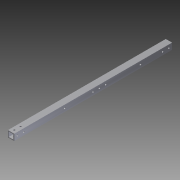
# Autodesk Inventor part: towermediumfrontthing
Saved by Autodesk Inventor 2011 SP1 (Build 150282100, 282)
## iProperties
Created: 2012-01-18
Part Number: towermediumfrontthing
Document SubType Name: Modeling
Designer: Christopher
Density: 1 g/cm^3
Author: Christopher
Autodesk Inventor part; units mm, degrees
ref_plane "YZ Plane" through (0, 0, 0) normal (1, 0, 0) x (0, 1, 0)
ref_plane "XZ Plane" through (0, 0, 0) normal (0, 1, 0) x (-1, 0, 0)
ref_plane "XY Plane" through (0, 0, 0) normal (0, 0, 1) x (1, 0, 0)
sketch "Sketch1" plane through (0, 0, 0) normal (0, 0, 1) x (1, 0, 0)
  line L0 (0, 0) -> (25.4, 0)
  line L1 (25.4, 0) -> (25.4, 25.4)
  line L2 (25.4, 25.4) -> (0, 25.4)
  line L3 (0, 25.4) -> (0, 0)
  line L4 (3.175, 3.175) -> (22.225, 3.175)
  line L5 (22.225, 3.175) -> (22.225, 22.225)
  line L6 (22.225, 22.225) -> (3.175, 22.225)
  line L7 (3.175, 22.225) -> (3.175, 3.175)
  dimension "d0" = 25.4
  dimension "d1" = 25.4
  dimension "d2" = 3.175
  constraints: 16 end point, 4 parallel, 2 perpendicular, 1 horizontal, 3 other
  measures "d0" distance of L1.end L2.end
  measures "d1" distance of L0.end L1.end
  measures "d2" distance between parallel lines of L3 L7
extrude "Extrusion1" add sketch "Sketch1" against normal blind 635
sketch "Sketch3" plane through (0, 25.4, 0) normal (0, 1, 0) x (1, 0, 0)
  line L0 (25.4, 0) -> (0, 0) projected
  point P0 (12.7, 12.7)
  point P1 (12.7, 38.1)
  dimension "d24" = 12.7
  dimension "d25" = 25.4
  measures "d24" distance from line of L0 point (12.7, 12.7)
  measures "d25" distance of point (12.7, 38.1) point (12.7, 12.7)
hole "Hole3" at (12.7, 25.4, -12.7) at (12.7, 25.4, -38.1) direction (0, -1, 0) diameter 6.35 depth 25.4 tip angle 118
sketch "Sketch4" plane through (0, 0, 0) normal (-1, 0, 0) x (0, 0, 1)
  line L0 (0, 25.4) -> (0, 0) projected
  point P0 (-12.7, 12.7)
  point P1 (-38.1, 12.7)
  dimension "d33" = 12.7
  dimension "d34" = 25.4
  measures "d33" distance from line of point (-12.7, 12.7) L0
  measures "d34" distance of point (-38.1, 12.7) point (-12.7, 12.7)
hole "Hole4" at (0, 12.7, -12.7) at (0, 12.7, -38.1) direction (1, 0, 0) diameter 6.35 depth 25.4 tip angle 118
sketch "Sketch5" plane through (25.4, 0, 0) normal (1, 0, 0) x (0, 0, -1)
  line L0 (0, 0) -> (0, 25.4) projected
  point P0 (317.5, 12.7)
  point P1 (342.9, 12.7)
  point P2 (368.3, 12.7)
  point P3 (596.9, 12.7)
  point P4 (622.3, 12.7)
  point P5 (647.7, 12.7)
  point P6 (812.8, 12.7)
  point P7 (508, 12.7)
  point P8 (203.2, 12.7)
  point P9 (977.9, 12.7)
  point P10 (952.5, 12.7)
  dimension "d42" = 317.5
  dimension "d43" = 25.4
  dimension "d44" = 25.4
  dimension "d45" = 25.4
  dimension "d46" = 25.4
  dimension "d47" = 228.6
  dimension "d55" = 165.1
  dimension "d56" = 139.7
  dimension "d57" = 114.3
  dimension "d58" = 25.4
  dimension "d59" = 139.7
  measures "d42" distance from line of point (317.5, 12.7) L0
  measures "d43" distance of point (342.9, 12.7) point (317.5, 12.7)
  measures "d44" distance of point (342.9, 12.7) point (368.3, 12.7)
  measures "d45" distance of point (622.3, 12.7) point (596.9, 12.7)
  measures "d46" distance of point (647.7, 12.7) point (622.3, 12.7)
  measures "d47" distance of point (368.3, 12.7) point (596.9, 12.7)
  measures "d55" distance of point (812.8, 12.7) point (647.7, 12.7)
  measures "d56" distance of point (368.3, 12.7) point (508, 12.7)
  measures "d57" distance of point (317.5, 12.7) point (203.2, 12.7)
  measures "d58" distance of point (977.9, 12.7) point (952.5, 12.7)
  measures "d59" distance of point (812.8, 12.7) point (952.5, 12.7)
hole "Hole5" at (25.4, 12.7, -317.5) at (25.4, 12.7, -342.9) at (25.4, 12.7, -368.3) at (25.4, 12.7, -596.9) at (25.4, 12.7, -622.3) at (25.4, 12.7, -647.7) at (25.4, 12.7, -203.2) at (25.4, 12.7, -508) at (25.4, 12.7, -812.8) at (25.4, 12.7, -952.5) at (25.4, 12.7, -977.9) direction (-1, 0, 0) diameter 6.35 depth 25.4 tip angle 118
body "Solid1"
